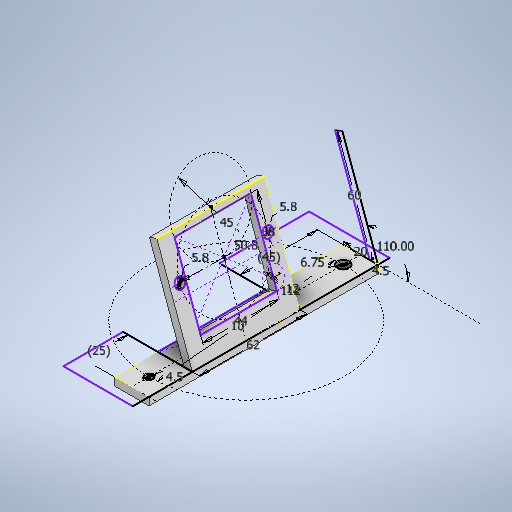
# Autodesk Inventor part: ThriftyCamMountTopSwerve
Saved by Autodesk Inventor 2025 (Build 290162000, 162)
## iProperties
Created: 2025-03-15
Part Number: ThriftyCamMountTopSwerve
Material: Generic
Document SubType Name: Modeling
Designer: john
Density: 1 g/cm^3
Appearance: Default
Author: john
Autodesk Inventor part; units mm, degrees
ref_plane "YZ Plane" through (0, 0, 0) normal (1, 0, 0) x (0, 1, 0)
ref_plane "XZ Plane" through (0, 0, 0) normal (0, 1, 0) x (-1, 0, 0)
ref_plane "XY Plane" through (0, 0, 0) normal (0, 0, 1) x (1, 0, 0)
sketch "Sketch1" plane through (0, 0, 0) normal (0, 0, 1) x (1, 0, 0)
  line L0 (-10, -2.25) -> (10, -2.25)
  line L1 (10, -2.25) -> (10, 2.25)
  line L2 (10, 2.25) -> (-10, 2.25)
  line L3 (-10, 2.25) -> (-10, -2.25)
  line L4 (-10, -2.25) -> (10, 2.25) construction
  line L5 (10, -2.25) -> (-10, 2.25) construction
  line L6 (10, 2.25) -> (-10.5212, 58.6316)
  line L7 (10, 2.25) -> (70, 2.25) construction
  line L8 (-10.5212, 58.6316) -> (-14.7498, 57.0925)
  line L9 (5.2112, 2.25) -> (-14.7498, 57.0925)
  point P0 (0, 0)
  dimension "d0" = 20
  dimension "d1" = 4.5
  dimension "d11" = 60
  dimension "d12" = 110
  constraints: 20 end point, 3 parallel, 2 horizontal, 2 midpoint, 1 equal length, 1 perpendicular, 1 point on line
  measures "d0" distance of L2.end L1.end
  measures "d1" distance of L1.end L0.end
  measures "d11" distance of L1.end L6.end
  measures "d12" angle of L7 L6
extrude "Extrusion1" add sketch "Sketch1" along normal blind 132 contours L3 L2 L1 L0
sketch "Sketch2" plane through (-10, 2.25, 0) normal (0, 1, 0) x (1, 0, 0)
  line L0 (20, -132) -> (0, -132) construction
  line L1 (10, -132) -> (10, 0) construction
  line L2 (20, 0) -> (0, 0) construction
  line L3 (0, 0) -> (0, -132) construction
  line L4 (0, -66) -> (20, -66) construction
  line L5 (20, 0) -> (20, -132) construction
  circle A0 centre (10, -66) radius 56 construction
  circle A1 centre (10, -122) radius 2.25
  circle A2 centre (10, -10) radius 3.375
  line L6 (0, -76) -> (20, -76) construction
  line L7 (0, -107) -> (20, -107)
  line L8 (20, -107) -> (20, -45)
  line L9 (20, -45) -> (0, -45)
  line L10 (0, -45) -> (0, -107)
  line L11 (0, -107) -> (20, -45) construction
  line L12 (20, -107) -> (0, -45) construction
  line L13 (20, -107) -> (-19.9682, -107)
  line L14 (-19.9682, -107) -> (-19.9682, -141.3538)
  line L15 (-19.9682, -141.3538) -> (20, -141.3538)
  line L16 (20, -141.3538) -> (20, -107)
  line L17 (20, -45) -> (-26.4005, -45)
  line L18 (-26.4005, -45) -> (-26.4005, 6.7001)
  line L19 (-26.4005, 6.7001) -> (20, 6.7001)
  line L20 (20, 6.7001) -> (20, -45)
  point P0 (10, -76)
  dimension "d4" = 112
  dimension "d5" = 4.5
  dimension "d6" = 6.75
  dimension "d9" = 10
  dimension "d10" = 62
  dimension "d16" = 25
  dimension "d17" = 45
  constraints: 34 end point, 7 midpoint, 7 parallel, 4 coincident, 4 perpendicular, 3 centre point, 3 horizontal, 3 point on line, 2 point on circle
  measures "d4" diameter of A0
  measures "d5" diameter of A1
  measures "d6" diameter of A2
  measures "d9" distance between parallel lines of L4 L6
  measures "d10" distance of L8.end L7.end
  measures "d16" distance between parallel lines of L0 L7
  measures "d17" distance between parallel lines of L2 L9
extrude "Extrusion2" cut sketch "Sketch2" against normal blind 132 contours A1 | A2
extrude "Extrusion3" add sketch "Sketch1" along normal blind 132 contours L2 L9 L8 L6
sketch "Sketch3" plane through (10, -2.25, 132) normal (1, 0, 0) x (0, 0, -1)
  point P0 (132, 2.25)
extrude "Extrusion4" cut sketch "Sketch2" along normal blind 132 contours A1 | A2 | L7 L16 L15 L14 L13 | L17 L18 L19 L20 L9
sketch "Sketch4" plane through (-10.5212, 58.6316, 107) normal (0.9396926, 0.3420201, 0) x (0, 0, -1)
  line L0 (62, 0) -> (0, 0) projected
  line L1 (31, 0) -> (31, -57.7119) construction
  line L2 (62, 0) -> (62, -58.3621) construction
  line L3 (62, -28.8559) -> (0, -28.8559) construction
  circle A0 centre (31, 0) radius 22.5 construction
  line L4 (62, -22.5) -> (0, -22.5) construction
  circle A1 centre (31, -22.5) radius 25.4 construction
  circle A2 centre (5.6, -22.5) radius 2.9
  circle A3 centre (56.4, -22.5) radius 2.9
  line L5 (9, -3.5) -> (53, -3.5)
  line L6 (53, -3.5) -> (53, -41.5)
  line L7 (53, -47.5) -> (9, -47.5)
  line L8 (9, -47.5) -> (9, -3.5)
  line L9 (9, -3.5) -> (53, -41.5) construction
  line L10 (53, -3.5) -> (9, -41.5) construction
  circle A4 centre (53, -41.5) radius 6 construction
  line L11 (53, -47.5) -> (53, -41.5)
  point P0 (107, -58.6941)
  point P1 (31, -28.8559)
  dimension "d20" = 45
  dimension "d28" = 12
  dimension "d21" = 50.8
  dimension "d22" = 5.8
  dimension "d23" = 5.8
  dimension "d26" = 44
  dimension "d27" = 38
  constraints: 20 end point, 4 midpoint, 4 point on line, 3 centre point, 3 coincident, 3 horizontal, 3 point on circle, 2 parallel, 2 perpendicular, 2 vertical alignment, 1 vertical, 4 other
  measures "d21" diameter of A1
  measures "d22" diameter of A2
  measures "d23" diameter of A3
  measures "d26" distance of L7.end L7.start
  measures "d27" distance of L6.end L5.end
extrude "Extrusion5" cut sketch "Sketch4" against normal blind 12 contours A2 | A3
extrude "Extrusion6" cut sketch "Sketch4" against normal blind 6 contours L5 L6 L11 L7 L8
body "Solid1"
